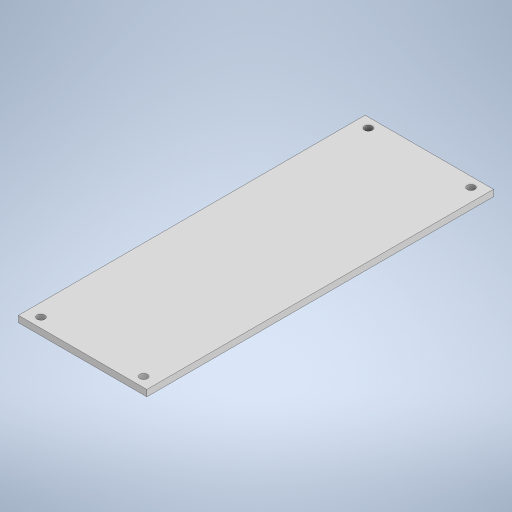
# Autodesk Inventor part: side_front
Saved by Autodesk Inventor 2024 (Build 280153000, 153)
## iProperties
Created: 2026-03-15
Part Number: side_front
Material: Generic
Document SubType Name: Modeling
Designer: HP
Density: 1 g/cm^3
Appearance: Default
Author: HP
Autodesk Inventor part; units mm, degrees
ref_plane "YZ Plane" through (0, 0, 0) normal (1, 0, 0) x (0, 1, 0)
ref_plane "XZ Plane" through (0, 0, 0) normal (0, 1, 0) x (-1, 0, 0)
ref_plane "XY Plane" through (0, 0, 0) normal (0, 0, 1) x (1, 0, 0)
sketch "Sketch1" plane through (0, 0, 0) normal (0, 1, 0) x (-1, 0, 0)
  line L0 (0, 0) -> (0, 135)
  line L1 (0, 135) -> (0, -135)
  line L2 (0, -135) -> (50, -135)
  line L3 (50, -135) -> (-50, -135)
  line L4 (-50, -135) -> (-50, 135)
  line L5 (-50, 135) -> (50, 135)
  line L6 (50, 135) -> (50, -135)
  line L7 (50, 135) -> (50, 127.5)
  line L8 (50, 127.5) -> (40, 127.5)
  circle A0 centre (40, 127.5) radius 3
  line L9 (40, 127.5) -> (-40, 127.5)
  circle A1 centre (-40, 127.5) radius 3
  line L10 (50, 0) -> (-50, 0)
  circle A2 centre (40, -127.5) radius 3
  circle A3 centre (-40, -127.5) radius 3
  dimension "d0" = 135
  dimension "d1" = 270
  dimension "d2" = 50
  dimension "d3" = 100
  dimension "d4" = 7.5
  dimension "d5" = 10
  dimension "d6" = 6
  dimension "d7" = 80
  dimension "d8" = 6
  constraints: 22 end point, 4 centre point, 4 perpendicular, 3 point on line, 2 coincident, 2 horizontal, 2 midpoint, 2 symmetric about line, 1 vertical, 2 other
  measures "d0" distance of L0.start L0.end
  measures "d1" distance of L0.end L1.end
  measures "d2" distance of L1.end L2.end
  measures "d3" distance of L2.end L3.end
  measures "d4" distance of L5.end L7.end
  measures "d5" distance of L7.end L8.end
  measures "d6" diameter of A0
  measures "d7" distance of L9.start L9.end
  measures "d8" diameter of A1
extrude "Extrusion1" add sketch "Sketch1" along normal blind 5 contours L10 L4 L5 L0 | L10 L6 L2 L1 | L0 L9 A0 L8 L6 L10 | L1 L3 L4 L10 | L0 L5 L6 L8 A0 L9
body "Solid1"
